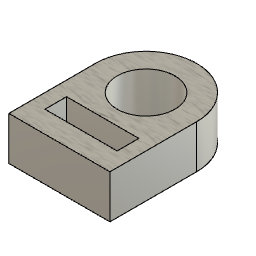
Solution 1 (Autodesk Fusion 360 design; units mm, degrees)
Autodesk Fusion 360 part; units mm, degrees
sketch "Sketch1" plane through (0, 0, 0) normal (0, 1, 0) x (1, 0, 0)
  line L0 (0, 0) -> (0, -60)
  line L1 (0, -60) -> (70, -60)
  line L2 (70, -60) -> (70, 0)
  arc A0 (70, 0) -> (0, 0) centre (35, 0) ccw
  line L3 (10, -30) -> (60, -30)
  line L4 (60, -30) -> (60, -45)
  line L5 (60, -45) -> (10, -45)
  line L6 (10, -45) -> (10, -30)
  circle A1 centre (35, 0) radius 20
  dimension "d1" = 60
  dimension "d2" = 70
  dimension "d5" = 50
  dimension "d6" = 15
  dimension "d7" = 40
  constraint coincident L0.start A0.end
  constraint vertical L0
  constraint perpendicular L0 L1
  constraint perpendicular L1 L2
  constraint horizontal L3
  constraint vertical L4
  constraint horizontal L5
  constraint vertical L6
  constraint concentric A0 A1
  measures "d1" distance of L0.start L0.end
  measures "d2" distance of L0.end L1.end
  measures "d5" distance of L3.start L3.end
  measures "d6" distance of L3.start L5.end
  measures "d7" diameter of A1
extrude "Extrude1" add sketch "Sketch1" along normal blind 10
extrude "Extrude2" add 1 faces at (43.3333, 10, 55) along direction (0, 1, 0) blind 20
